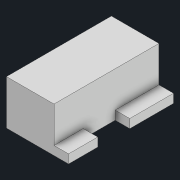
# Autodesk Inventor part: AC-DC transformer
Saved by Autodesk Inventor 2022 (Build 260153000, 153)
## iProperties
Created: 2022-01-12
Part Number: AC-DC transformer
Material: Generic
Document SubType Name: Modeling
Designer: Andres
Density: 1 g/cm^3
Appearance: Default
Author: Andres
Autodesk Inventor part; units mm, degrees
ref_plane "YZ Plane" through (0, 0, 0) normal (1, 0, 0) x (0, 1, 0)
ref_plane "XZ Plane" through (0, 0, 0) normal (0, 1, 0) x (-1, 0, 0)
ref_plane "XY Plane" through (0, 0, 0) normal (0, 0, 1) x (1, 0, 0)
sketch "Sketch1" plane through (0, 0, 0) normal (0, 1, 0) x (-1, 0, 0)
  line L0 (16.3, 0) -> (0, 0)
  line L1 (0, 0) -> (0, -36)
  line L2 (0, -36) -> (16.3, -36)
  line L3 (16.3, -36) -> (16.3, 0)
  dimension "d0" = 36
  dimension "d1" = 16.3
  constraints: 8 end point, 2 parallel, 1 coincident, 1 horizontal, 1 perpendicular
  measures "d0" distance of L2.end L0.start
  measures "d1" distance of L0.start L0.end
extrude "Extrusion1" add sketch "Sketch1" along normal blind 15.3
sketch "Sketch2" plane through (0, 0, 0) normal (1, 0, 0) x (0, 0, -1)
  line L0 (0, 0) -> (0, 15.3) projected
  line L1 (0, 0) -> (10, 0)
  line L2 (10, 0) -> (10, 3)
  line L3 (10, 3) -> (0, 3)
  line L4 (0, 3) -> (0, 0)
  line L5 (0, 0) -> (36, 0) projected
  line L6 (36, 0) -> (21, 0)
  line L7 (21, 0) -> (21, 3)
  line L8 (21, 3) -> (36, 3)
  line L9 (36, 3) -> (36, 0)
  point P0 (0, 3)
  dimension "d4" = 10
  dimension "d5" = 3
  dimension "d6" = 15
  constraints: 16 end point, 4 parallel, 2 horizontal, 2 perpendicular, 1 collinear
  measures "d4" distance of L2.end L3.end
  measures "d5" distance of L1.end L2.end
  measures "d6" distance of L7.end L8.end
extrude "Extrusion2" add sketch "Sketch2" along normal blind 5
body "Solid1"
